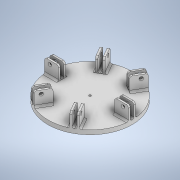
# Autodesk Inventor part: outer_hub
Saved by Autodesk Inventor 2020 (Build 240168000, 168)
## iProperties
Created: 2019-09-24
Part Number: outer_hub
Material: Generic
Document SubType Name: Modeling
Designer: dlr6513
Density: 1 g/cm^3
Appearance: Default
Author: dlr6513
Autodesk Inventor part; units mm, degrees
ref_plane "YZ Plane" through (0, 0, 0) normal (1, 0, 0) x (0, 1, 0)
ref_plane "XZ Plane" through (0, 0, 0) normal (0, 1, 0) x (-1, 0, 0)
ref_plane "XY Plane" through (0, 0, 0) normal (0, 0, 1) x (1, 0, 0)
sketch "Sketch1" plane through (0, 0, 0) normal (0, 1, 0) x (-1, 0, 0)
  circle A0 centre (0, 0) radius 60
  circle A1 centre (0, 0) radius 1.5
  line L0 (40, -2.5) -> (40, -5)
  line L1 (40, -5) -> (59.7913, -5)
  line L2 (40, 2.5) -> (40, 5)
  line L3 (40, 5) -> (59.7913, 5)
  line L4 (40, -2.5) -> (59.9479, -2.5)
  line L5 (40, 2.5) -> (59.9479, 2.5)
  line L6 (15.6699, 37.141) -> (25.5655, 54.2808)
  line L7 (17.8349, 35.891) -> (27.8089, 53.1664)
  line L8 (17.8349, 35.891) -> (15.6699, 37.141)
  line L9 (22.1651, 33.391) -> (32.139, 50.6664)
  line L10 (24.3301, 32.141) -> (34.2258, 49.2808)
  line L11 (22.1651, 33.391) -> (24.3301, 32.141)
  line L12 (-24.3301, 32.141) -> (-34.2258, 49.2808)
  line L13 (-22.1651, 33.391) -> (-32.139, 50.6664)
  line L14 (-22.1651, 33.391) -> (-24.3301, 32.141)
  line L15 (-17.8349, 35.891) -> (-27.8089, 53.1664)
  line L16 (-15.6699, 37.141) -> (-25.5655, 54.2808)
  line L17 (-17.8349, 35.891) -> (-15.6699, 37.141)
  line L18 (-40, -5) -> (-59.7913, -5)
  line L19 (-40, -2.5) -> (-59.9479, -2.5)
  line L20 (-40, -2.5) -> (-40, -5)
  line L21 (-40, 2.5) -> (-59.9479, 2.5)
  line L22 (-40, 5) -> (-59.7913, 5)
  line L23 (-40, 2.5) -> (-40, 5)
  line L24 (-15.6699, -37.141) -> (-25.5655, -54.2808)
  line L25 (-17.8349, -35.891) -> (-27.8089, -53.1664)
  line L26 (-17.8349, -35.891) -> (-15.6699, -37.141)
  line L27 (-22.1651, -33.391) -> (-32.139, -50.6664)
  line L28 (-24.3301, -32.141) -> (-34.2258, -49.2808)
  line L29 (-22.1651, -33.391) -> (-24.3301, -32.141)
  line L30 (24.3301, -32.141) -> (34.2258, -49.2808)
  line L31 (22.1651, -33.391) -> (32.139, -50.6664)
  line L32 (22.1651, -33.391) -> (24.3301, -32.141)
  line L33 (17.8349, -35.891) -> (27.8089, -53.1664)
  line L34 (15.6699, -37.141) -> (25.5655, -54.2808)
  line L35 (17.8349, -35.891) -> (15.6699, -37.141)
  point P0 (60, -5)
  point P1 (60, 5)
  point P2 (60, -2.5)
  point P3 (60, 2.5)
  dimension "d0" = 120
  dimension "d1" = 3
  dimension "d8" = 360
  constraints: 72 end point, 4 point on circle, 2 centre point, 2 coincident, 85 other
  measures "d0" diameter of A0
  measures "d1" diameter of A1
extrude "Extrusion1" add sketch "Sketch1" along normal blind 6 contours A0 L4 L0 L1 L30 L32 L31 L33 L35 L34 L24 L26 L25 L27 L29 L28 L18 L20 L19 L21 L23 L22 L12 L14 L13 L15 L17 L16 L6 L8 L7 L9 L11 L10 L3 L2 L5
extrude "Extrusion2" add sketch "Sketch1" along normal blind 26 contours L5 L2 L3 A0 | A0 L1 L0 L4 | L10 L11 L9 A0 | A0 L31 L32 L30 | L7 L8 L6 A0 | A0 L34 L35 L33 | L16 L17 L15 A0 | A0 L25 L26 L24 | L13 L14 L12 A0 | A0 L28 L29 L27 | L22 L23 L21 A0 | A0 L19 L20 L18
sketch "Sketch2" plane through (-15.6699, 6, 37.141) normal (0.8660254, 0, 0.5) x (0.5, 0, -0.8660254)
  circle A0 centre (-12.2913, 15) radius 2.5
  line L0 (-19.7913, 20) -> (0, 20) projected
  line L1 (-19.7913, 0) -> (-19.7913, 20) projected
  point P0 (40, -6)
  dimension "d14" = 5
  dimension "d15" = 5
  dimension "d16" = 7.5
  constraints: 1 centre point
  measures "d14" diameter of A0
  measures "d15" distance from line of L0 A0.centre
  measures "d16" distance from line of L1 A0.centre
extrude "Extrusion3" cut sketch "Sketch2" against normal through all
sketch "Sketch3" plane through (-59.7913, 6, 5) normal (0, 0, 1) x (1, 0, 0)
  circle A0 centre (7.5, 15) radius 2.5
  line L0 (0, 20) -> (19.7913, 20) projected
  line L1 (0, 0) -> (0, 20) projected
  point P0 (59.7913, -6)
  dimension "d19" = 5
  dimension "d20" = 5
  dimension "d21" = 7.5
  constraints: 1 centre point
  measures "d19" diameter of A0
  measures "d20" distance from line of L0 A0.centre
  measures "d21" distance from line of L1 A0.centre
extrude "Extrusion4" cut sketch "Sketch3" against normal through all
sketch "Sketch4" plane through (-24.3301, 6, -32.141) normal (-0.8660254, 0, 0.5) x (0.5, 0, 0.8660254)
  circle A0 centre (-12.2913, 15) radius 2.5
  line L0 (-19.7913, 20) -> (0, 20) projected
  line L1 (-19.7913, 0) -> (-19.7913, 20) projected
  point P0 (40, -6)
  dimension "d24" = 5
  dimension "d25" = 5
  dimension "d26" = 7.5
  constraints: 1 centre point
  measures "d24" diameter of A0
  measures "d25" distance from line of L0 A0.centre
  measures "d26" distance from line of L1 A0.centre
extrude "Extrusion5" cut sketch "Sketch4" against normal through all
sketch "Sketch5" plane through (15.6699, 6, -37.141) normal (-0.8660254, 0, -0.5) x (-0.5, 0, 0.8660254)
  circle A0 centre (-12.2913, 15) radius 2.5
  line L0 (-19.7913, 0) -> (-19.7913, 20) projected
  line L1 (-19.7913, 20) -> (0, 20) projected
  point P0 (40, -6)
  dimension "d29" = 5
  dimension "d30" = 7.5
  dimension "d31" = 5
  constraints: 1 centre point
  measures "d29" diameter of A0
  measures "d30" distance from line of L0 A0.centre
  measures "d31" distance from line of L1 A0.centre
extrude "Extrusion6" cut sketch "Sketch5" against normal through all
sketch "Sketch6" plane through (59.7913, 6, -5) normal (0, 0, -1) x (-1, 0, 0)
  circle A0 centre (7.5, 15) radius 2.5
  line L0 (0, 20) -> (19.7913, 20) projected
  line L1 (0, 0) -> (0, 20) projected
  point P0 (59.7913, -6)
  dimension "d34" = 5
  dimension "d35" = 5
  dimension "d36" = 7.5
  constraints: 1 centre point
  measures "d34" diameter of A0
  measures "d35" distance from line of L0 A0.centre
  measures "d36" distance from line of L1 A0.centre
extrude "Extrusion7" cut sketch "Sketch6" against normal through all
sketch "Sketch7" plane through (24.3301, 6, 32.141) normal (0.8660254, 0, -0.5) x (-0.5, 0, -0.8660254)
  circle A0 centre (-12.2913, 15) radius 2.5
  line L0 (-19.7913, 20) -> (0, 20) projected
  line L1 (-19.7913, 0) -> (-19.7913, 20) projected
  point P0 (40, -6)
  dimension "d39" = 5
  dimension "d40" = 5
  dimension "d41" = 7.5
  constraints: 1 centre point
  measures "d39" diameter of A0
  measures "d40" distance from line of L0 A0.centre
  measures "d41" distance from line of L1 A0.centre
extrude "Extrusion8" cut sketch "Sketch7" against normal through all
fillet "Fillet1" radius 3.175 24 edges at (33.1896, 26, 49.9845) (26.693, 26, 53.7353) (16.7524, 26, 36.516) (23.2476, 26, 32.766) (-26.693, 26, 53.7353) (-33.1896, 26, 49.9845) (-16.7524, 26, 36.516) (-23.2476, 26, 32.766) (-40, 26, -3.75) (-40, 26, 3.75) (-59.8826, 26, -3.7508) (-59.8826, 26, 3.7508) (-33.1896, 26, -49.9845) (-23.2476, 26, -32.766) (-26.693, 26, -53.7353) (-16.7524, 26, -36.516) (33.1896, 26, -49.9845) (26.693, 26, -53.7353) (16.7524, 26, -36.516) (23.2476, 26, -32.766) (59.8826, 26, -3.7508) (59.8826, 26, 3.7508) (40, 26, 3.75) (40, 26, -3.75)
fillet "Fillet2" radius 2.54 24 edges at (-20.6177, 6, 45.7109) (-22.8219, 6, 44.5287) (-27.152, 6, 42.0287) (20.6177, 6, 45.7109) (-29.278, 6, 40.7109) (-49.8957, 6, 5) (-49.9739, 6, 2.5) (-49.9739, 6, -2.5) (-49.8957, 6, -5) (-29.278, 6, -40.7109) (-27.152, 6, -42.0287) (-22.8219, 6, -44.5287) (-20.6177, 6, -45.7109) (20.6177, 6, -45.7109) (22.8219, 6, -44.5287) (27.152, 6, -42.0287) (29.278, 6, -40.7109) (49.8957, 6, -5) (49.9739, 6, -2.5) (49.9739, 6, 2.5) (49.8957, 6, 5) (29.278, 6, 40.7109) (27.152, 6, 42.0287) (22.8219, 6, 44.5287)
body "Solid1"
